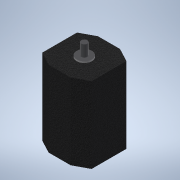
# Autodesk Inventor part: motor
Saved by Autodesk Inventor 2021 (Build 250183000, 183)
## iProperties
Created: 2022-04-14
Part Number: motor
Material: Stahl
Document SubType Name: Modeling
Designer: 10154704
Density: 7.85 g/cm^3
Appearance: Stahl
Author: 10154704
Autodesk Inventor part; units mm, degrees
ref_plane "YZ Plane" through (0, 0, 0) normal (1, 0, 0) x (0, 1, 0)
ref_plane "XZ Plane" through (0, 0, 0) normal (0, 1, 0) x (-1, 0, 0)
ref_plane "XY Plane" through (0, 0, 0) normal (0, 0, 1) x (1, 0, 0)
sketch "Skizze1" plane through (0, 0, 0) normal (0, 0, 1) x (1, 0, 0)
  line L0 (-32.5, 32.5) -> (32.5, 32.5)
  line L1 (32.5, 32.5) -> (32.5, -32.5)
  line L2 (32.5, -32.5) -> (-32.5, -32.5)
  line L3 (-32.5, -32.5) -> (-32.5, 32.5)
  point P0 (0, 0)
  point P1 (-32.5, 16.5982)
  point P2 (-16.4712, 32.5)
  dimension "d0" = 65
  dimension "d1" = 65
  dimension "d2" = 32.5
  dimension "d3" = 32.5
  constraints: 8 end point, 2 parallel, 2 point on line, 1 horizontal, 1 perpendicular
  measures "d0" distance between parallel lines of L1 L3
  measures "d1" distance between parallel lines of L2 L0
  measures "d2" distance from line of L1 point (0, 0)
  measures "d3" distance from line of L0 point (0, 0)
extrude "Extrusion1" add sketch "Skizze1" along normal blind 100
sketch "Skizze2" plane through (0, 0, 100) normal (0, 0, 1) x (1, 0, 0)
  circle A0 centre (0, 0) radius 10
  dimension "d6" = 20
  constraints: 1 centre point, 1 coincident
  measures "d6" diameter of A0
extrude "Extrusion2" add sketch "Skizze2" along normal blind 2
sketch "Skizze3" plane through (0, 0, 102) normal (0, 0, 1) x (1, 0, 0)
  circle A0 centre (0, 0) radius 4
  dimension "d9" = 8
  constraints: 1 centre point, 1 coincident
  measures "d9" diameter of A0
extrude "Extrusion3" add sketch "Skizze3" along normal blind 15
sketch "Sketch4" plane through (0, 0, 100) normal (0, 0, 1) x (1, 0, 0)
  line L0 (32.5, 32.5) -> (-32.5, 32.5) projected
  line L1 (-14.5, 32.5) -> (-32.5, 22.9292)
  line L2 (-32.5, 32.5) -> (-32.5, -32.5) projected
  line L3 (-32.5, 32.5) -> (-14.5, 32.5)
  line L4 (-32.5, 32.5) -> (-32.5, 22.9292)
  point P0 (0, 0)
  dimension "d15" = 28
  dimension "d16" = 18
  constraints: 6 end point, 2 point on line, 1 horizontal, 1 perpendicular
  measures "d15" angle of L0 L1
  measures "d16" distance from line of L2 L1.start
extrude "Extrusion4" cut sketch "Sketch4" against normal up to surface (100 mm away)
mirror "Mirror1" about plane through (0, 0, 0) normal (1, 0, 0) of "Extrusion4"
mirror "Mirror2" about plane through (0, 0, 0) normal (0, 1, 0) of "Extrusion4", "Mirror1"
sketch "Sketch5" plane through (0, 0, 0) normal (1, 0, 0) x (0, 1, 0)
  line L0 (32.5, 0) -> (32.5, 100) projected
  line L1 (32.5, 20.5) -> (36.5, 20.5)
  line L2 (36.5, 20.5) -> (36.5, 22.5)
  line L3 (36.5, 22.5) -> (40.3063, 22.5)
  line L4 (47.5, 30) -> (32.5, 30)
  line L5 (32.5, 20.5) -> (32.5, 30)
  line L6 (22.9292, 0) -> (32.5, 0) projected
  arc A0 (40.3063, 22.5) -> (47.5, 27) centre (40.3063, 30.5) ccw
  line L7 (47.5, 27) -> (47.5, 30)
  point P0 (0, 0)
  dimension "d19" = 4
  dimension "d20" = 2
  dimension "d21" = 15
  dimension "d22" = 30
  dimension "d23" = 15
  dimension "d24" = 8
  dimension "d25" = 3
  constraints: 12 end point, 3 perpendicular, 2 point on circle, 2 point on line, 1 centre point, 1 collinear, 1 horizontal, 1 tangent, 1 vertical
  measures "d19" distance between parallel lines of L0 L2
  measures "d20" distance between parallel lines of L3 L1
  measures "d21" diameter of L3 L4
  measures "d22" distance between parallel lines of L6 L4
  measures "d23" distance between parallel lines of L0 L7
  measures "d24" radius of A0
  measures "d25" distance of L7.start L4.start
revolve "Revolution1" add sketch "Sketch5" angle 360 about axis through (0, 47.5, 30) along (0, -1, 0)
equation "\"d1\" = d0"
equation "\"d2\" = 0.5 * d0"
equation "\"d3\" = 0.5 * d1"
